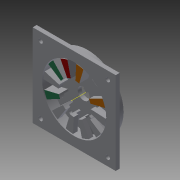
# Autodesk Inventor part: bayonet container 12
Saved by Autodesk Inventor 2015 (Build 190159000, 159)
## iProperties
Created: 2014-09-09
Part Number: bayonet container 12
Material: Generic
Document SubType Name: Modeling
Designer: ericd_000
Density: 1 g/cm^3
Appearance: Default
Author: ericd_000
Autodesk Inventor part; units mm, degrees
ref_plane "YZ Plane" through (0, 0, 0) normal (1, 0, 0) x (0, 1, 0)
ref_plane "XZ Plane" through (0, 0, 0) normal (0, 1, 0) x (-1, 0, 0)
ref_plane "XY Plane" through (0, 0, 0) normal (0, 0, 1) x (1, 0, 0)
sketch "Sketch1" plane through (0, 0, 0) normal (0, 1, 0) x (-1, 0, 0)
  line L0 (52.5, 52.5) -> (-52.5, 52.5)
  line L1 (-52.5, 52.5) -> (-52.5, -52.5)
  line L2 (-52.5, -52.5) -> (52.5, -52.5)
  line L3 (52.5, -52.5) -> (52.5, 52.5)
  circle A0 centre (0, 0) radius 35
  circle A1 centre (42.5, 42.5) radius 2.75
  circle A2 centre (-42.5, 42.5) radius 2.75
  circle A3 centre (-42.5, -42.5) radius 2.75
  circle A4 centre (42.5, -42.5) radius 2.75
  point P0 (52.5, 0)
  point P1 (0, -52.5)
  dimension "d0" = 105
  dimension "d1" = 105
  dimension "d2" = 70
  dimension "d3" = 5.5
  dimension "d4" = 10
  dimension "d5" = 10
  dimension "d8" = 360
  constraints: 8 end point, 5 centre point, 2 midpoint, 2 parallel, 1 coincident, 1 horizontal, 1 horizontal alignment, 1 perpendicular, 1 vertical alignment, 9 other
  measures "d0" distance of L2.end L0.start
  measures "d1" distance of L1.end L2.end
  measures "d2" diameter of A0
  measures "d3" diameter of A1
  measures "d4" distance from line of L3 A1.centre
  measures "d5" distance from line of L0 A1.centre
extrude "Extrusion1" add sketch "Sketch1" along normal blind 5
sketch "Sketch2" plane through (0, 0, 0) normal (0, -1, 0) x (1, 0, 0)
  circle A0 centre (0, 0) radius 45.5
  dimension "d12" = 91
  constraints: 1 centre point, 1 coincident
  measures "d12" diameter of A0
extrude "Extrusion2" cut sketch "Sketch2" against normal blind 10
sketch "Sketch3" plane through (0, 0, 0) normal (0, -1, 0) x (1, 0, 0)
  circle A0 centre (0, 0) radius 45.5
  circle A1 centre (0, 0) radius 40.5
  dimension "d15" = 91
  dimension "d16" = 81
  constraints: 2 centre point, 2 coincident
  measures "d15" diameter of A0
  measures "d16" diameter of A1
extrude "Extrusion3" add sketch "Sketch3" against normal blind 17
sketch "Sketch4" plane through (0, 17, 0) normal (0, 1, 0) x (1, 0, 0)
  circle A0 centre (0, 0) radius 40.5
  point P0 (0, 0)
  dimension "d42" = 81
  constraints: 1 centre point, 1 coincident
  measures "d42" diameter of A0
extrude "Extrusion4" add sketch "Sketch4" against normal blind 5
sketch "Sketch5" plane through (0, 12, 0) normal (0, -1, 0) x (1, 0, 0)
  circle A0 centre (0, 33) radius 2.5
  line L0 (0, 0) -> (0, 33) construction
  dimension "d21" = 5
  dimension "d117" = 33
  constraints: 2 end point, 1 centre point, 1 vertical
  measures "d21" diameter of A0
  measures "d117" distance of L0.start L0.end
extrude "Extrusion5" cut sketch "Sketch5" against normal through all
pattern_circular "Circular Pattern1" count 12 over 360 about axis through (0, 0, 0) along (0, 1, 0) of "Extrusion5"
sketch "Sketch6" plane through (0, 12, 0) normal (0, -1, 0) x (1, 0, 0)
  circle A0 centre (0, 0) radius 7.5
  point P0 (0, 0)
  dimension "d28" = 15
  constraints: 1 centre point, 1 coincident
  measures "d28" diameter of A0
extrude "Extrusion6" cut sketch "Sketch6" against normal blind 10
sketch "Sketch7" plane through (0, 12, 0) normal (0, -1, 0) x (1, 0, 0)
  circle A0 centre (0, 0) radius 20.5
  circle A1 centre (0, 0) radius 40.5 projected
  line L0 (0, 0) -> (-13.3071, -15.594) construction
  circle A2 centre (-16.5, -28.5788) radius 2.5 projected
  line L1 (0, 0) -> (-14.8642, -14.1176) construction
  circle A3 centre (0, 0) radius 39.5
  line L2 (-14.8642, -14.1176) -> (-28.6407, -27.2022)
  line L3 (-13.3071, -15.594) -> (-25.6404, -30.0469)
  point P0 (-25.8631, 31.1664)
  point P1 (-29.3658, -27.8908)
  dimension "d31" = 20
  dimension "d43" = 81
  dimension "d44" = 79
  dimension "d45" = 19
  dimension "d66" = 6
  dimension "d67" = 174
  constraints: 8 end point, 6 point on circle, 2 centre point, 2 coincident, 2 collinear, 1 point on line
  measures "d31" radial gap between concentric circles of A1 A0
  measures "d43" diameter of A1
  measures "d44" diameter of A3
  measures "d45" radial gap between concentric circles of A3 A0
  measures "d66" distance from line of L3 A2.centre
  measures "d67" angle of L2 L3
extrude "Extrusion7" add sketch "Sketch7" along normal blind 11.5 contours A0 L3 A3 L2 picked at (-22.7302, -24.1463)
sketch "Sketch9" plane through (0, 0.5, 0) normal (0, -1, 0) x (1, 0, 0)
  circle A0 centre (0, 0) radius 29.9834
  circle A1 centre (0, 0) radius 39.9778
  line L0 (0, 0) -> (-26.8767, 13.2908) construction
  line L1 (-35.8356, 17.721) -> (-26.8767, 13.2908)
  point P0 (0, 0)
  constraints: 4 end point, 2 coincident, 1 collinear, 1 point on line, 6 other
sketch "Sketch10" plane through (-13.3071, 0.5, -15.594) normal (0.7606815, 0, -0.6491252) x (-0.6491252, 0, -0.7606815)
  line L0 (0, 0) -> (19, 0)
  line L1 (19, 0) -> (19, 5.75)
  line L2 (19, 11.5) -> (19, 0) projected
  line L3 (0, 11.5) -> (0, 0) projected
  line L4 (0, 5.75) -> (19, 5.75)
  line L5 (0, 11.5) -> (19, 11.5)
  line L6 (-20.5, -3.9) -> (-20.5, 19.9) projected
  point P0 (-20.5, -0.5)
  dimension "d46" = 5.75
  constraints: 8 end point, 2 horizontal, 2 midpoint, 1 parallel
  measures "d46" distance between parallel lines of L0 L4
revolve "Revolution2" add sketch "Sketch10" angle 7.5 about axis through (0, 0, 0) along (0, -1, 0) contours L3 L4 L1 L0
pattern_circular "Circular Pattern2" count 12 over 360 about axis through (0, 0, 0) along (0, 1, 0) of "Extrusion7", "Revolution2"
sketch "Sketch13" plane through (0, 17, 0) normal (0, 1, 0) x (1, 0, 0)
  circle A0 centre (0, 0) radius 45.5
  circle A1 centre (0, 0) radius 41.5
  dimension "d52" = 4
  dimension "d53" = 91
  constraints: 2 centre point, 2 coincident
  measures "d52" radial gap between concentric circles of A0 A1
  measures "d53" diameter of A0
extrude "Extrusion10" add sketch "Sketch13" along normal blind 13
sketch "Sketch17" plane through (0, 0, 0) normal (0, 0, 1) x (1, 0, 0)
  line L0 (41.5, 17) -> (-41.5, 17) projected
  line L1 (70, 17) -> (-70, 17)
  line L2 (-70, 17) -> (-70, 47.3289)
  line L3 (-70, 47.3289) -> (70, 47.3289)
  line L4 (70, 47.3289) -> (70, 17)
  line L5 (-52.5, 0) -> (52.5, 0) projected
  point P0 (0, 0)
  point P1 (0, 47.3289)
  point P2 (0, 0)
  dimension "d116" = 140
  constraints: 8 end point, 2 midpoint, 2 parallel, 1 horizontal, 1 perpendicular, 1 point on line, 1 vertical alignment
  measures "d116" distance of L2.end L3.end
extrude "Extrusion13" cut sketch "Sketch17" along normal through all both and the other way through all
sketch "Sketch14" plane through (0, 30, 0) normal (0, 1, 0) x (1, 0, 0)
  circle A0 centre (0, 0) radius 65
  constraints: 1 centre point, 1 coincident
extrude "Extrusion11" add sketch "Sketch14" along normal blind 5
sketch "Sketch18" plane through (0, 17, 0) normal (0, 1, 0) x (1, 0, 0)
  point P0 (0, 0)
sketch "Sketch21" plane through (0, 0, 0) normal (0, 0, 1) x (1, 0, 0)
  line L0 (79.7641, 55.8787) -> (-85.0233, 55.8787)
  line L1 (-85.0233, 55.8787) -> (-85.0233, 20)
  line L2 (-85.0233, 20) -> (79.7641, 20)
  line L3 (79.7641, 20) -> (79.7641, 55.8787)
  point P0 (0, 0)
  constraints: 8 end point, 2 parallel, 1 horizontal, 1 perpendicular
extrude "Extrusion17" cut sketch "Sketch21" along normal through all both and the other way through all
sketch "Sketch26" plane through (0, 12, 0) normal (0, -1, 0) x (1, 0, 0)
  circle A0 centre (-22.985, 30.0089) radius 1.5
  line L0 (-27.2022, 28.6407) -> (-14.1176, 14.8642) projected
  point P0 (0, 0)
  point P1 (-14.1176, 14.8642)
  point P2 (13.9968, 38.0045)
  point P3 (0.1327, 34.8029)
  dimension "d95" = 3
  dimension "d97" = 4
  dimension "d101" = 37.8
  constraints: 1 centre point, 1 other
  measures "d95" diameter of A0
  measures "d101" distance of point (0, 0) A0.centre
extrude "Extrusion20" cut sketch "Sketch26" against normal blind 10
sketch "Sketch27" plane through (0, 12, 0) normal (0, -1, 0) x (1, 0, 0)
  circle A0 centre (-22.985, 30.0089) radius 2.5
  circle A1 centre (-22.985, 30.0089) radius 1.5 projected
  point P0 (0, 0)
  dimension "d100" = 5
  constraints: 1 centre point, 1 concentric
  measures "d100" diameter of A0
extrude "Extrusion21" cut sketch "Sketch27" against normal blind 3
pattern_circular "Circular Pattern4" count 2 over 360 about axis through (0, 0, 0) along (0, 1, 0) of "Extrusion20", "Extrusion21"
sketch "Sketch29" plane through (33.1366, 0.5, -21.4992) normal (0.544283, 0, 0.8389017) x (0.8389017, 0, -0.544283)
  line L0 (-19, 0) -> (0, 0) projected
  line L1 (-19, 0) -> (-16, 0)
  line L2 (-16, 0) -> (-16, 5.75)
  line L3 (-16, 5.75) -> (-19, 5.75)
  line L4 (-19, 5.75) -> (-19, 0)
  line L5 (0, 5.75) -> (-19, 5.75) projected
  point P0 (-39.5, -0.5)
  point P1 (-13.5, 0)
  point P2 (-18.3771, 0)
  dimension "d115" = 3
  constraints: 8 end point, 2 parallel, 1 collinear, 1 horizontal, 1 perpendicular
  measures "d115" distance between parallel lines of L4 L2
extrude "Extrusion23" add sketch "Sketch29" along normal blind 2
body "Solid1"
